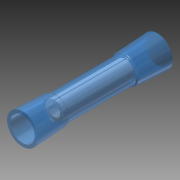
# Autodesk Inventor part: 16-14 double sided femal tube heat shrink
Saved by Autodesk Inventor 2014 (Build 180170000, 170)
## iProperties
Created: 2013-07-21
Part Number: 16-14 double sided femal tube heat shrink
Material: Generic
Document SubType Name: Modeling
Designer: Saville
Mass: 0.578492 g
Surface Area: 15.7572 cm^2
Volume: 0.578492 cm^3
Density: 1 g/cm^3
Appearance: Default
Author: Saville
Autodesk Inventor part; units mm, degrees
ref_plane "YZ Plane" through (0, 0, 0) normal (1, 0, 0) x (0, 1, 0)
ref_plane "XZ Plane" through (0, 0, 0) normal (0, 1, 0) x (-1, 0, 0)
ref_plane "XY Plane" through (0, 0, 0) normal (0, 0, 1) x (1, 0, 0)
sketch "Sketch1" plane through (0, 0, 0) normal (0, 0, 1) x (1, 0, 0)
  circle A0 centre (0, 0) radius 2.921
  dimension "d0" = 5.842
  constraints: 1 centre point, 1 coincident
  measures "d0" diameter of A0
extrude "Extrusion1" add sketch "Sketch1" along normal mid plane 16.51
sketch "Sketch2" plane through (0, 0, 8.255) normal (0, 0, 1) x (1, 0, 0)
  circle A0 centre (0, 0) radius 2.921 construction
  circle A1 centre (0, 0) radius 3.2512
  dimension "d3" = 6.5024
  constraints: 1 centre point, 1 coincident
  measures "d3" diameter of A1
extrude "Extrusion2" add sketch "Sketch2" along normal blind 7.7724 draft 3
fillet "Fillet1" radius 0.508 2 edges at (-2.921, 0, 8.255) (-3.2512, 0, 8.255)
mirror "Mirror1" about plane through (0, 0, 0) normal (0, 0, 1) of "Extrusion2", "Fillet1"
shell "Shell1" thickness 0.762 removed faces 2 at (1.0171, -0.0499, 16.0274) at (1.0171, -0.0499, -16.0274)
sketch "Sketch3" plane through (0, 0, 0) normal (0, 1, 0) x (-1, 0, 0)
  arc A0 (-3.2648, 8.515) -> (-3.0933, 8.1604) centre (-2.7575, 8.5416) ccw projected
  line L0 (-3.2648, 8.515) -> (-3.6585, 16.0274) projected
  line L1 (-3.6585, 16.0274) -> (-2.8955, 16.0274) projected
  line L2 (-2.8955, 16.0274) -> (-2.5091, 8.6547) projected
  arc A1 (-2.159, 7.7791) -> (-2.5091, 8.6547) centre (-3.429, 7.7791) ccw projected
  line L3 (-2.159, 7.7791) -> (-2.159, -7.7791) projected
  arc A2 (-2.5091, -8.6547) -> (-2.159, -7.7791) centre (-3.429, -7.7791) ccw projected
  line L4 (-2.5091, -8.6547) -> (-2.8955, -16.0274) projected
  line L5 (-2.8955, -16.0274) -> (-3.6585, -16.0274) projected
  line L6 (-3.6585, -16.0274) -> (-3.2648, -8.515) projected
  arc A3 (-3.0933, -8.1604) -> (-3.2648, -8.515) centre (-2.7575, -8.5416) ccw projected
  arc A4 (-3.0933, -8.1604) -> (-2.921, -7.7791) centre (-3.429, -7.7791) ccw projected
  line L7 (-2.921, -7.7791) -> (-2.921, 7.7791) projected
  arc A5 (-2.921, 7.7791) -> (-3.0933, 8.1604) centre (-3.429, 7.7791) ccw projected
  arc A6 (3.0933, 8.1604) -> (3.2648, 8.515) centre (2.7575, 8.5416) ccw projected
  arc A7 (3.0933, 8.1604) -> (2.921, 7.7791) centre (3.429, 7.7791) ccw projected
  line L8 (2.921, 7.7791) -> (2.921, -7.7791) projected
  arc A8 (2.921, -7.7791) -> (3.0933, -8.1604) centre (3.429, -7.7791) ccw projected
  arc A9 (3.2648, -8.515) -> (3.0933, -8.1604) centre (2.7575, -8.5416) ccw projected
  line L9 (3.2648, -8.515) -> (3.6585, -16.0274) projected
  line L10 (3.6585, -16.0274) -> (2.8955, -16.0274) projected
  line L11 (2.8955, -16.0274) -> (2.5091, -8.6547) projected
  arc A10 (2.159, -7.7791) -> (2.5091, -8.6547) centre (3.429, -7.7791) ccw projected
  line L12 (2.159, -7.7791) -> (2.159, 7.7791) projected
  arc A11 (2.5091, 8.6547) -> (2.159, 7.7791) centre (3.429, 7.7791) ccw projected
  line L13 (2.5091, 8.6547) -> (2.8955, 16.0274) projected
  line L14 (2.8955, 16.0274) -> (3.6585, 16.0274) projected
  line L15 (3.6585, 16.0274) -> (3.2648, 8.515) projected
  line L16 (1.3589, -8.4415) -> (2.159, -8.4415)
  line L17 (2.159, -8.4415) -> (2.159, 8.4415)
  line L18 (2.159, 8.4415) -> (1.3589, 8.4415)
  line L19 (1.3589, 8.4415) -> (1.3589, -8.4415)
  line L20 (0, 0) -> (5.4328, 0) construction
  line L21 (0, -22.4384) -> (0, 22.4384) projected
  dimension "d8" = 0.8001
  constraints: 10 end point, 2 parallel, 2 perpendicular, 1 collinear, 1 horizontal, 1 other
  measures "d8" distance between parallel lines of L19 L17
revolve "Revolution1" add sketch "Sketch3" angle 360 about axis through (0, 0, -10) along (0, 0, 1) separate body contours L12 L17 L16 L19 L18
sketch "Sketch4" plane through (0, 0, 8.4415) normal (0, 0, 1) x (1, 0, 0)
  circle A0 centre (0, 0) radius 1.3589 projected
  circle A1 centre (0, 0) radius 2.159 projected
  line L0 (0, 0) -> (0, 3.9072) construction
  line L1 (-0.1168, 2.1558) -> (-0.1168, 1.3539)
  line L2 (0.1168, 2.1558) -> (0.1168, 1.3539)
  constraints: 6 end point, 4 point on circle, 2 parallel, 1 vertical, 1 other
extrude "Extrusion3" cut sketch "Sketch4" against normal through all contours A0 L1 A1 L2 picked at (0.0909, 1.6227) bodies 2
body "Solid1"
body "Solid2"
